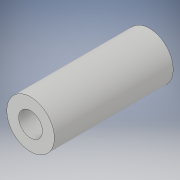
# Autodesk Inventor part: 1''_spacer
Saved by Autodesk Inventor 2018 (Build 220112000, 112)
## iProperties
Created: 2018-07-13
Part Number: 1''_spacer
Material: Generic
Document SubType Name: Modeling
Designer: baoan
Density: 1 g/cm^3
Appearance: Default
Author: baoan
Autodesk Inventor part; units mm, degrees
ref_plane "YZ Plane" through (0, 0, 0) normal (1, 0, 0) x (0, 1, 0)
ref_plane "XZ Plane" through (0, 0, 0) normal (0, 1, 0) x (-1, 0, 0)
ref_plane "XY Plane" through (0, 0, 0) normal (0, 0, 1) x (1, 0, 0)
sketch "Sketch1" plane through (0, 0, 0) normal (0, 0, 1) x (1, 0, 0)
  circle A0 centre (0, 0) radius 2.54
  circle A1 centre (0, 0) radius 5.08
  dimension "d0" = 5.08
  dimension "d1" = 10.16
  constraints: 2 centre point, 2 coincident
  measures "d0" diameter of A0
  measures "d1" diameter of A1
extrude "Extrusion1" add sketch "Sketch1" along normal mid plane 25.4
body "Solid1"
